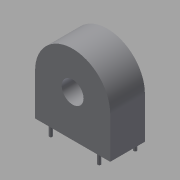
# Autodesk Inventor part: cr8348-1000
Saved by Autodesk Inventor 2013 (Build 170138000, 138)
## iProperties
Created: 2014-06-07
Part Number: cr8348-1000
Material: Generic
Document SubType Name: Modeling
Designer: Brad
Density: 1 g/cm^3
Author: Brad
Autodesk Inventor part; units mm, degrees
ref_plane "YZ Plane" through (0, 0, 0) normal (1, 0, 0) x (0, 1, 0)
ref_plane "XZ Plane" through (0, 0, 0) normal (0, 1, 0) x (-1, 0, 0)
ref_plane "XY Plane" through (0, 0, 0) normal (0, 0, 1) x (1, 0, 0)
sketch "Sketch1" plane through (0, 0, 0) normal (0, 0, 1) x (1, 0, 0)
  circle A0 centre (0, 0) radius 3.429
  arc A1 (11.811, 0) -> (-11.811, 0) centre (0, 0) ccw
  line L0 (11.811, 0) -> (11.811, -13.081)
  line L1 (11.811, -13.081) -> (-11.811, -13.081)
  line L2 (-11.811, -13.081) -> (-11.811, 0)
  dimension "d0" = 6.858
  dimension "d2" = 23.622
  dimension "d3" = 13.081
  dimension "d4" = 13.081
  constraints: 6 end point, 2 centre point, 2 coincident, 2 point on circle, 2 tangent, 1 perpendicular, 1 vertical
  measures "d0" diameter of A0
  measures "d2" diameter of A1
  measures "d3" distance from line of A1.centre L1
  measures "d4" distance of L1.end L2.end
extrude "Extrusion1" add sketch "Sketch1" against normal blind 10.922
sketch "Sketch2" plane through (-11.811, -13.081, 0) normal (0, -1, 0) x (1, 0, 0)
  line L0 (0, 0) -> (0, -10.922) projected
  line L1 (23.622, -10.922) -> (0, -10.922) projected
  circle A0 centre (4.191, -0.762) radius 0.508
  circle A1 centre (2.286, -10.16) radius 0.508
  circle A2 centre (21.336, -10.16) radius 0.508
  circle A3 centre (19.431, -0.762) radius 0.508
  point P0 (11.811, 0)
  dimension "d7" = 1.016
  dimension "d9" = 1.016
  dimension "d10" = 1.016
  dimension "d11" = 1.016
  dimension "d12" = 15.24
  dimension "d13" = 9.398
  dimension "d14" = 9.398
  dimension "d15" = 19.05
  dimension "d16" = 1.905
  dimension "d18" = 0
  dimension "d19" = 1.905
  dimension "d20" = 2.286
  dimension "d21" = 0.762
  constraints: 4 centre point
  measures "d7" diameter of A0
  measures "d9" diameter of A1
  measures "d10" diameter of A2
  measures "d11" diameter of A3
  measures "d12" distance of A3.centre A0.centre
  measures "d13" vertical distance of A2.centre A3.centre
  measures "d14" vertical distance of A0.centre A1.centre
  measures "d15" distance between centres of A2 A1
  measures "d16" horizontal distance of A1.centre A0.centre
  measures "d18" vertical distance of A3.centre A0.centre
  measures "d19" horizontal distance of A2.centre A3.centre
  measures "d20" distance from line of L0 A1.centre
  measures "d21" distance from line of L1 A1.centre
extrude "Extrusion2" add sketch "Sketch2" along normal blind 3.048
body "Solid1"
